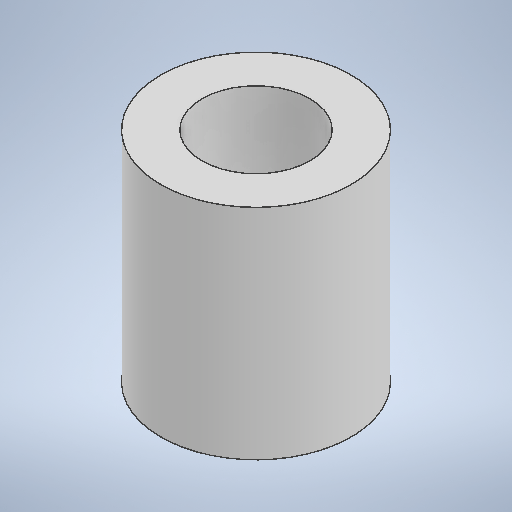
# Autodesk Inventor part: Printed Standoff 6.9mm
Saved by Autodesk Inventor 2025 (Build 290162000, 162)
## iProperties
Created: 2025-04-20
Part Number: Printed Standoff 6.9mm
Material: Generic
Document SubType Name: Modeling
Designer: User
Density: 1 g/cm^3
Appearance: Default
Author: User
Autodesk Inventor part; units mm, degrees
ref_plane "YZ Plane" through (0, 0, 0) normal (1, 0, 0) x (0, 1, 0)
ref_plane "XZ Plane" through (0, 0, 0) normal (0, 1, 0) x (-1, 0, 0)
ref_plane "XY Plane" through (0, 0, 0) normal (0, 0, 1) x (1, 0, 0)
sketch "Sketch1" plane through (0, 0, 0) normal (0, 1, 0) x (-1, 0, 0)
  circle A0 centre (0, 0) radius 3
  circle A1 centre (0, 0) radius 1.7
  dimension "d0" = 6
  dimension "d3" = 3.4
  constraints: 2 centre point, 2 coincident
  measures "d0" diameter of A0
  measures "d3" diameter of A1
extrude "Extrusion1" add sketch "Sketch1" along normal blind 6.9 contours A0 | A1
extrude "Extrusion2" cut sketch "Sketch1" along normal blind 3.1 contours A1
sketch "Sketch2" plane through (0, 6.9, 0) normal (0, 1, 0) x (1, 0, 0)
  circle A0 centre (0, 0) radius 1.7 projected
extrude "Extrusion3" cut sketch "Sketch2" against normal blind 3.1
sketch "Sketch3" plane through (0, 3.8, 0) normal (0, 1, 0) x (1, 0, 0)
  line L0 (1, 2) -> (-1, 2)
  line L1 (-1, 2) -> (-1, -2)
  line L2 (-1, -2) -> (1, -2)
  line L3 (1, -2) -> (1, 2)
  line L4 (1, 2) -> (-1, -2) construction
  line L5 (-1, 2) -> (1, -2) construction
  circle A0 centre (0, 0) radius 1.7 projected
  point P0 (1, -1.3748)
  point P1 (1, 1.3748)
  point P2 (-1, 1.3748)
  point P3 (-1, -1.3748)
  dimension "d8" = 2
  constraints: 12 end point, 2 midpoint, 2 parallel, 1 horizontal, 1 perpendicular
  measures "d8" distance of L2.end L1.end
extrude "Extrusion4" cut sketch "Sketch3" against normal blind 0.2 contours L3 A0 L1
sketch "Sketch4" plane through (0, 3.1, 0) normal (0, -1, 0) x (1, 0, 0)
  line L0 (1, -1.3748) -> (1, 1.3748) projected
  arc A0 (-1, -1.3748) -> (1, -1.3748) centre (0, 0) ccw projected
  line L1 (-1, 1.3748) -> (-1, -1.3748) projected
  arc A1 (1, 1.3748) -> (-1, 1.3748) centre (0, 0) ccw projected
extrude "Extrusion5" cut sketch "Sketch4" against normal blind 0.2
body "Solid1"
